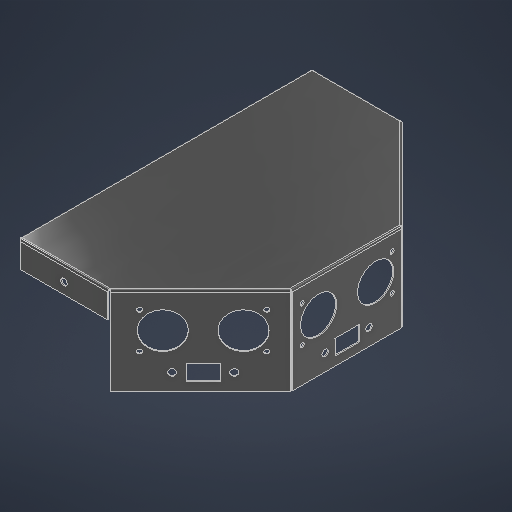
# Autodesk Inventor part: saxuravi
Saved by Autodesk Inventor 2026.2 (Build 302298000, 298)
## iProperties
Created: 2026-03-09
Part Number: saxuravi
Material: Generic
Document SubType Name: Sheet Metal
Designer: User
Density: 1 g/cm^3
Sheet Metal Rule: Default_mm
Appearance: Dark Gray
Flat Pattern Width: 13.3262 cm
Flat Pattern Length: 18.8754 cm
Flat Pattern Area: 251.537 cm^2
Sheet Metal Width: 133.262 mm
Sheet Metal Length: 188.754 mm
Sheet Metal Area: 25153.694 mm^2
Author: User
Autodesk Inventor part; units mm, degrees
ref_plane "YZ Plane" through (0, 0, 0) normal (1, 0, 0) x (0, 1, 0)
ref_plane "XZ Plane" through (0, 0, 0) normal (0, 1, 0) x (-1, 0, 0)
ref_plane "XY Plane" through (0, 0, 0) normal (0, 0, 1) x (1, 0, 0)
sketch "Sketch1" plane through (0, 0, 0) normal (0, 1, 0) x (-1, 0, 0)
  line L0 (0, 0) -> (81, 0)
  line L1 (81, 0) -> (81, -132)
  line L2 (81, -132) -> (0, -132)
  line L3 (0, -132) -> (0, 0)
  dimension "d0" = 81
  dimension "d1" = 132
  measures "d0" distance of L1.end L2.end
  measures "d1" distance of L0.end L1.end
extrude "Plate1" add sketch "Sketch1" along normal blind 0.5
chamfer "Corner Chamfer1" distance 41 angle 45 2 edges at (0, 0.25, 0) (0, 0.25, -132)
sketch "Sketch2" plane through (-40.6464, -0.5, 0.3536) normal (0.7071068, 0, 0.7071068) x (0, 1, 0)
  line L0 (0, -57.9828) -> (0, 0)
  line L1 (0, 0) -> (-39, 0)
  line L2 (-39, 0) -> (-39, -57.9828)
  line L3 (-39, -57.9828) -> (0, -57.9828)
  constraints: 6 end point, 1 horizontal, 1 perpendicular, 1 vertical
edge flange "Flange1" height 40 angle 90 thickness 0.5 bend radius 0.5 thickness toward (0.7071068, 0, 0.7071068) relief tear relief width 0.5 relief depth 0.25 edges at (-20.5, 0, -20.5) wall of the first edge with corners at (0.3536, -0.5, -40.6464) (-40.6464, -0.5, 0.3536) (-40.6464, -39.5, 0.3536) (0.3536, -39.5, -40.6464)
bend "Bend1"
corner "Corner1"
sketch "Sketch3" plane through (0.5, -0.5, -41) normal (1, 0, 0) x (0, 1, 0)
  line L0 (0, -50) -> (0, 0)
  line L1 (0, 0) -> (-39, 0)
  line L2 (-39, 0) -> (-39, -50)
  line L3 (-39, -50) -> (0, -50)
  constraints: 6 end point, 1 horizontal, 1 perpendicular, 1 vertical
edge flange "Flange2" height 40 angle 90 thickness 0.5 bend radius 0.5 thickness toward (1, 0, 0) relief tear relief width 0.5 relief depth 0.25 edges at (0, 0, -66) wall of the first edge with corners at (0.5, -0.5, -91) (0.5, -0.5, -41) (0.5, -39.5, -41) (0.5, -39.5, -91)
bend "Bend2"
corner "Corner2"
sketch "Sketch4" plane through (0.3536, -0.5, -91.3536) normal (0.7071068, 0, -0.7071068) x (0, 1, 0)
  line L0 (0, -57.9828) -> (0, 0)
  line L1 (0, 0) -> (-39, 0)
  line L2 (-39, 0) -> (-39, -57.9828)
  line L3 (-39, -57.9828) -> (0, -57.9828)
  constraints: 6 end point, 1 horizontal, 1 perpendicular, 1 vertical
edge flange "Flange3" height 40 angle 90 thickness 0.5 bend radius 0.5 thickness toward (0.7071068, 0, -0.7071068) relief tear relief width 0.5 relief depth 0.25 edges at (-20.5, 0, -111.5) wall of the first edge with corners at (-40.6464, -0.5, -132.3536) (0.3536, -0.5, -91.3536) (0.3536, -39.5, -91.3536) (-40.6464, -39.5, -132.3536)
bend "Bend3"
corner "Corner3"
sketch "Sketch5" plane through (-81, -0.5, 0.5) normal (0, 0, 1) x (1, 0, 0)
  line L0 (40, 0) -> (0, 0)
  line L1 (0, 0) -> (0, -11)
  line L2 (0, -11) -> (40, -11)
  line L3 (40, -11) -> (40, 0)
  constraints: 6 end point, 1 horizontal, 1 perpendicular, 1 vertical
edge flange "Flange4" height 12 angle 90 thickness 0.5 bend radius 0.5 thickness toward (0, 0, 1) relief tear relief width 0.5 relief depth 0.25 corner gap 0.5 corner form 0 edges at (-61, 0, 0) (-61, 0, -132) wall of the first edge with corners at (-41, -0.5, 0.5) (-81, -0.5, 0.5) (-81, -11.5, 0.5) (-41, -11.5, 0.5)
bend "Bend4"
corner "Corner4"
sketch "Sketch6" plane through (-81.5, -0.5, -132) normal (-1, 0, 0) x (0, -1, 0)
  line L0 (0, 132) -> (0, 0)
  line L1 (0, 0) -> (11, 0)
  line L2 (11, 0) -> (11, 132)
  line L3 (11, 132) -> (0, 132)
  constraints: 6 end point, 1 horizontal, 1 perpendicular, 1 vertical
edge flange "Flange5" height 12 angle 90 thickness 0.5 bend radius 0.5 thickness toward (-1, 0, 0) relief tear relief width 0.5 relief depth 0.25 edges at (-81, 0, -66) wall of the first edge with corners at (-81.5, -0.5, 0) (-81.5, -0.5, -132) (-81.5, -11.5, -132) (-81.5, -11.5, 0)
bend "Bend5"
corner "Corner5"
sketch "Sketch7" plane through (-40.2929, -39.5, 0.7071) normal (0.7071068, 0, 0.7071068) x (0.7071068, 0, -0.7071068)
  line L0 (0, 0) -> (0, 39) projected
  line L1 (57.9828, 0) -> (57.9828, 39) projected
  line L2 (0, 0) -> (57.9828, 0)
  line L3 (57.9828, 0) -> (57.9828, 39)
  line L4 (57.9828, 39) -> (0, 39)
  line L5 (0, 39) -> (0, 0)
  line L6 (7.5, 14) -> (52.5, 14)
  line L7 (52.5, 14) -> (52.5, 34)
  line L8 (52.5, 34) -> (7.5, 34)
  line L9 (7.5, 34) -> (7.5, 14)
  circle A0 centre (9.5, 32.25) radius 1
  circle A1 centre (50.5, 32.25) radius 1
  circle A2 centre (50.5, 15.75) radius 1
  circle A3 centre (9.5, 15.75) radius 1
  circle A4 centre (17, 24) radius 8.25
  circle A5 centre (43, 24) radius 8.25
  line L10 (7.5, 24) -> (52.5, 24)
  circle A6 centre (20, 7.5) radius 1.5
  circle A7 centre (40, 7.5) radius 1.5
  line L11 (24.5, 4) -> (35.5, 4)
  line L12 (35.5, 4) -> (35.5, 11)
  line L13 (35.5, 11) -> (24.5, 11)
  line L14 (24.5, 11) -> (24.5, 4)
  point P0 (28.9914, 39.5)
  point P1 (28.9914, 0)
  dimension "d56" = 45
  dimension "d57" = 20
  dimension "d58" = 5
  dimension "d59" = 7.5
  dimension "d60" = 2
  dimension "d61" = 2
  dimension "d62" = 2
  dimension "d63" = 1.75
  dimension "d64" = 2
  dimension "d65" = 41
  dimension "d66" = 1.75
  dimension "d67" = 16.5
  dimension "d68" = 2
  dimension "d69" = 2
  dimension "d70" = 16.5
  dimension "d71" = 2
  dimension "d72" = 16.5
  dimension "d73" = 16.5
  dimension "d74" = 26
  dimension "d75" = 10
  dimension "d76" = 10
  dimension "d77" = 9.5
  dimension "d129" = 3
  dimension "d130" = 3
  dimension "d131" = 11
  dimension "d132" = 7
  dimension "d133" = 20
  dimension "d134" = 4
  dimension "d135" = 3.5
  dimension "d136" = 3.5
  dimension "d137" = 20
  dimension "d138" = 24.5
  constraints: 26 end point, 8 centre point, 6 parallel, 3 horizontal, 3 midpoint, 3 perpendicular
  measures "d56" distance of L8.end L7.end
  measures "d57" distance of L7.end L6.end
  measures "d58" distance between parallel lines of L8 L4
  measures "d59" distance between parallel lines of L0 L9
  measures "d60" diameter of A0
  measures "d61" diameter of A1
  measures "d62" diameter of A2
  measures "d63" distance from line of L8 A0.centre
  measures "d64" distance from line of L9 A0.centre
  measures "d65" distance of A0.centre A1.centre
  measures "d66" distance from line of L8 A1.centre
  measures "d67" distance of A2.centre A1.centre
  measures "d68" distance from line of L7 A2.centre
  measures "d69" diameter of A3
  measures "d70" distance of A3.centre A0.centre
  measures "d71" distance from line of L9 A3.centre
  measures "d72" diameter of A4
  measures "d73" diameter of A5
  measures "d74" distance of A5.centre A4.centre
  measures "d75" distance from line of L8 A4.centre
  measures "d76" distance from line of L8 A5.centre
  measures "d77" distance from line of L9 A4.centre
  measures "d129" diameter of A6
  measures "d130" diameter of A7
  measures "d131" distance of L13.end L12.end
  measures "d132" distance of L12.end L11.end
  measures "d133" distance of A7.centre A6.centre
  measures "d134" distance from line of point (28.991, 0) L11
  measures "d135" distance from line of L11 A6.centre
  measures "d136" distance from line of L11 A7.centre
  measures "d137" distance from line of L5 A6.centre
  measures "d138" distance between parallel lines of L0 L14
sketch "Sketch10" plane through (0.7071, -39.5, -91.7071) normal (0.7071068, 0, -0.7071068) x (-0.7071068, 0, -0.7071068)
  line L0 (0, 0) -> (57.9828, 0)
  line L1 (57.9828, 0) -> (57.9828, 39)
  line L2 (57.9828, 39) -> (0, 39)
  line L3 (0, 39) -> (0, 0)
  line L4 (7.5, 14) -> (52.5, 14)
  line L5 (52.5, 14) -> (52.5, 34)
  line L6 (52.5, 34) -> (7.5, 34)
  line L7 (7.5, 34) -> (7.5, 14)
  circle A0 centre (9.5, 32.25) radius 1
  circle A1 centre (50.5, 32.25) radius 1
  circle A2 centre (50.5, 15.75) radius 1
  circle A3 centre (9.5, 15.75) radius 1
  circle A4 centre (17, 24) radius 8.25
  circle A5 centre (43, 24) radius 8.25
  line L8 (7.5, 24) -> (52.5, 24)
  circle A6 centre (20, 7.5) radius 1.5
  circle A7 centre (40, 7.5) radius 1.5
  line L9 (24.5, 4) -> (35.5, 4)
  line L10 (35.5, 4) -> (35.5, 11)
  line L11 (35.5, 11) -> (24.5, 11)
  line L12 (24.5, 11) -> (24.5, 4)
  point P0 (28.9914, 39.5)
  point P1 (28.9914, 0)
  dimension "d139" = 45
  dimension "d140" = 20
  dimension "d141" = 5
  dimension "d143" = 2
  dimension "d144" = 2
  dimension "d145" = 2
  dimension "d146" = 1.75
  dimension "d147" = 2
  dimension "d148" = 41
  dimension "d149" = 1.75
  dimension "d150" = 16.5
  dimension "d151" = 2
  dimension "d152" = 2
  dimension "d153" = 16.5
  dimension "d154" = 2
  dimension "d155" = 16.5
  dimension "d156" = 16.5
  dimension "d157" = 26
  dimension "d158" = 10
  dimension "d159" = 10
  dimension "d160" = 9.5
  dimension "d161" = 3
  dimension "d162" = 3
  dimension "d163" = 11
  dimension "d164" = 7
  dimension "d165" = 20
  dimension "d166" = 4
  dimension "d167" = 3.5
  dimension "d168" = 3.5
  dimension "d169" = 20
  constraints: 26 end point, 8 centre point, 6 parallel, 3 horizontal, 3 midpoint, 3 perpendicular
  measures "d139" distance of L6.end L5.end
  measures "d140" distance of L5.end L4.end
  measures "d141" distance between parallel lines of L6 L2
  measures "d143" diameter of A0
  measures "d144" diameter of A1
  measures "d145" diameter of A2
  measures "d146" distance from line of L6 A0.centre
  measures "d147" distance from line of L7 A0.centre
  measures "d148" distance of A0.centre A1.centre
  measures "d149" distance from line of L6 A1.centre
  measures "d150" distance of A2.centre A1.centre
  measures "d151" distance from line of L5 A2.centre
  measures "d152" diameter of A3
  measures "d153" distance of A3.centre A0.centre
  measures "d154" distance from line of L7 A3.centre
  measures "d155" diameter of A4
  measures "d156" diameter of A5
  measures "d157" distance of A5.centre A4.centre
  measures "d158" distance from line of L6 A4.centre
  measures "d159" distance from line of L6 A5.centre
  measures "d160" distance from line of L7 A4.centre
  measures "d161" diameter of A6
  measures "d162" diameter of A7
  measures "d163" distance of L11.end L10.end
  measures "d164" distance of L10.end L9.end
  measures "d165" distance of A7.centre A6.centre
  measures "d166" distance from line of point (28.991, 0) L9
  measures "d167" distance from line of L9 A6.centre
  measures "d168" distance from line of L9 A7.centre
  measures "d169" distance from line of L3 A6.centre
sketch "Sketch11" plane through (1, -39.5, -41) normal (1, 0, 0) x (0, 0, -1)
  line L0 (0, 0) -> (57.9828, 0)
  line L1 (57.9828, 0) -> (57.9828, 39)
  line L2 (57.9828, 39) -> (0, 39)
  line L3 (0, 39) -> (0, 0)
  line L4 (2.5, 14) -> (47.5, 14)
  line L5 (47.5, 14) -> (47.5, 34)
  line L6 (47.5, 34) -> (2.5, 34)
  line L7 (2.5, 34) -> (2.5, 14)
  circle A0 centre (4.5, 32.25) radius 1
  circle A1 centre (45.5, 32.25) radius 1
  circle A2 centre (45.5, 15.75) radius 1
  circle A3 centre (4.5, 15.75) radius 1
  circle A4 centre (12, 24) radius 8.25
  circle A5 centre (38, 24) radius 8.25
  line L8 (2.5, 24) -> (47.5, 24)
  circle A6 centre (15, 7.5) radius 1.5
  circle A7 centre (35, 7.5) radius 1.5
  line L9 (19.5, 4) -> (30.5, 4)
  line L10 (30.5, 4) -> (30.5, 11)
  line L11 (30.5, 11) -> (19.5, 11)
  line L12 (19.5, 11) -> (19.5, 4)
  point P0 (28.9914, 39.5)
  point P1 (28.9914, 0)
  dimension "d171" = 45
  dimension "d172" = 20
  dimension "d173" = 5
  dimension "d175" = 2
  dimension "d176" = 2
  dimension "d177" = 2
  dimension "d178" = 1.75
  dimension "d179" = 2
  dimension "d180" = 41
  dimension "d181" = 1.75
  dimension "d182" = 16.5
  dimension "d183" = 2
  dimension "d184" = 2
  dimension "d185" = 16.5
  dimension "d186" = 2
  dimension "d187" = 16.5
  dimension "d188" = 16.5
  dimension "d189" = 26
  dimension "d190" = 10
  dimension "d191" = 10
  dimension "d192" = 9.5
  dimension "d193" = 3
  dimension "d194" = 3
  dimension "d195" = 11
  dimension "d196" = 7
  dimension "d197" = 20
  dimension "d198" = 4
  dimension "d199" = 3.5
  dimension "d200" = 3.5
  dimension "d201" = 15
  dimension "d203" = 2.5
  dimension "d204" = 19.5
  constraints: 26 end point, 8 centre point, 6 parallel, 3 horizontal, 3 midpoint, 3 perpendicular
  measures "d171" distance of L6.end L5.end
  measures "d172" distance of L5.end L4.end
  measures "d173" distance between parallel lines of L6 L2
  measures "d175" diameter of A0
  measures "d176" diameter of A1
  measures "d177" diameter of A2
  measures "d178" distance from line of L6 A0.centre
  measures "d179" distance from line of L7 A0.centre
  measures "d180" distance of A0.centre A1.centre
  measures "d181" distance from line of L6 A1.centre
  measures "d182" distance of A2.centre A1.centre
  measures "d183" distance from line of L5 A2.centre
  measures "d184" diameter of A3
  measures "d185" distance of A3.centre A0.centre
  measures "d186" distance from line of L7 A3.centre
  measures "d187" diameter of A4
  measures "d188" diameter of A5
  measures "d189" distance of A5.centre A4.centre
  measures "d190" distance from line of L6 A4.centre
  measures "d191" distance from line of L6 A5.centre
  measures "d192" distance from line of L7 A4.centre
  measures "d193" diameter of A6
  measures "d194" diameter of A7
  measures "d195" distance of L11.end L10.end
  measures "d196" distance of L10.end L9.end
  measures "d197" distance of A7.centre A6.centre
  measures "d198" distance from line of point (28.991, 0) L9
  measures "d199" distance from line of L9 A6.centre
  measures "d200" distance from line of L9 A7.centre
  measures "d201" distance from line of L3 A6.centre
  measures "d203" distance between parallel lines of L3 L7
  measures "d204" distance between parallel lines of L3 L12
extrude "Cut4" cut sketch "Sketch7" against normal blind 0.5 contours L10 A4 | A4 L10 | L10 A5 | A5 L10 | A0 | A1 | A2 | A3 | A6 | A7 | L14 L13 L12 L11
extrude "Cut5" cut sketch "Sketch11" against normal blind 0.5 contours L8 A4 | A4 L8 | L8 A5 | A5 L8 | A0 | A1 | A2 | A3 | A6 | A7 | L12 L11 L10 L9
extrude "Cut6" cut sketch "Sketch10" against normal blind 0.5 contours L8 A4 | A4 L8 | L8 A5 | A5 L8 | A0 | A1 | A2 | A3 | A6 | A7 | L12 L11 L10 L9
sketch "Sketch12" plane through (-81, -11.5, 1) normal (0, 0, 1) x (1, 0, 0)
  circle A0 centre (20, 5) radius 1.5
  line L0 (40, 11) -> (0, 11) projected
  line L1 (40, 11) -> (40, 0) projected
  point P0 (81, 11.5)
  dimension "d211" = 3
  dimension "d212" = 6
  dimension "d213" = 20
  constraints: 1 centre point
  measures "d211" diameter of A0
  measures "d212" distance from line of L0 A0.centre
  measures "d213" distance from line of L1 A0.centre
sketch "Sketch13" plane through (-41, -11.5, -133) normal (0, 0, -1) x (-1, 0, 0)
  circle A0 centre (20, 5) radius 1.5
  line L0 (40, 11) -> (0, 11) projected
  line L1 (40, 11) -> (40, 0) projected
  point P0 (-41, 11.5)
  dimension "d214" = 3
  dimension "d215" = 6
  dimension "d216" = 20
  constraints: 1 centre point
  measures "d214" diameter of A0
  measures "d215" distance from line of L0 A0.centre
  measures "d216" distance from line of L1 A0.centre
extrude "Cut7" cut sketch "Sketch13" against normal blind 0.5
extrude "Cut8" cut sketch "Sketch12" against normal blind 0.5
sketch "Sketch14" plane through (-82, -11.5, -132) normal (-1, 0, 0) x (0, 0, 1)
  circle A0 centre (41, 5) radius 1.5
  line L0 (91, -28) -> (91, 11) projected
  circle A1 centre (91, 5) radius 1.5
  line L1 (132, 11) -> (0, 11) projected
  point P0 (132, 11.5)
  dimension "d221" = 3
  dimension "d222" = 3
  dimension "d223" = 6
  dimension "d224" = 50
  dimension "d225" = 6
  constraints: 2 centre point, 1 point on line
  measures "d221" diameter of A0
  measures "d222" diameter of A1
  measures "d223" distance from line of L1 A1.centre
  measures "d224" distance of A0.centre A1.centre
  measures "d225" distance from line of L1 A0.centre
extrude "Cut9" cut sketch "Sketch14" against normal blind 0.5
equation "\"d205\" = Thickness"
equation "\"d207\" = Thickness"
equation "\"d209\" = Thickness"
equation "\"d217\" = Thickness"
equation "\"d219\" = Thickness"
equation "\"d226\" = Thickness"
equation "\"d2\" = Thickness"
equation "\"d6\" = BendReliefWidth"
equation "\"d7\" = BendReliefDepth"
equation "\"d8\" = MinimumRemnant"
equation "\"d9\" = TransitionRadius"
equation "\"d12\" = BendRadius"
equation "\"d13\" = CornerReliefSize"
equation "\"d14\" = GapSize"
equation "\"d15\" = JacobiRadiusSize"
equation "\"d16\" = BendReliefWidth"
equation "\"d17\" = BendReliefDepth"
equation "\"d18\" = MinimumRemnant"
equation "\"d19\" = TransitionRadius"
equation "\"d22\" = BendRadius"
equation "\"d23\" = CornerReliefSize"
equation "\"d24\" = GapSize"
equation "\"d25\" = JacobiRadiusSize"
equation "\"d26\" = BendReliefWidth"
equation "\"d27\" = BendReliefDepth"
equation "\"d28\" = MinimumRemnant"
equation "\"d29\" = TransitionRadius"
equation "\"d32\" = BendRadius"
equation "\"d33\" = CornerReliefSize"
equation "\"d34\" = GapSize"
equation "\"d35\" = JacobiRadiusSize"
equation "\"d36\" = BendReliefWidth"
equation "\"d37\" = BendReliefDepth"
equation "\"d38\" = MinimumRemnant"
equation "\"d39\" = TransitionRadius"
equation "\"d42\" = BendRadius"
equation "\"d43\" = CornerReliefSize"
equation "\"d44\" = GapSize"
equation "\"d45\" = JacobiRadiusSize"
equation "\"d46\" = BendReliefWidth"
equation "\"d47\" = BendReliefDepth"
equation "\"d48\" = MinimumRemnant"
equation "\"d49\" = TransitionRadius"
equation "\"d52\" = BendRadius"
equation "\"d53\" = CornerReliefSize"
equation "\"d54\" = GapSize"
equation "\"d55\" = JacobiRadiusSize"
equation "\"BendRadius\" = Thickness"
equation "\"BendReliefWidth\" = Thickness"
equation "\"BendReliefDepth\" = 0.5 * Thickness"
equation "\"CornerReliefSize\" = 4 * Thickness"
equation "\"MinimumRemnant\" = 2 * Thickness"
equation "\"TransitionRadius\" = BendRadius"
equation "\"JacobiRadiusSize\" = BendRadius"
equation "\"GapSize\" = Thickness"
equation "\"Thickness\" = 0.5"
body "Solid1"
